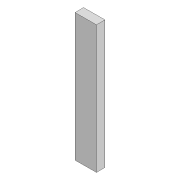
# Autodesk Inventor part: simple_object2
Saved by Autodesk Inventor 2021 (Build 250183000, 183)
## iProperties
Created: 2022-04-11
Part Number: simple_object2
Material: Generic
Document SubType Name: Modeling
Designer: Derm
Density: 1 g/cm^3
Appearance: Default
Author: Derm
Autodesk Inventor part; units mm, degrees
ref_plane "YZ Plane" through (0, 0, 0) normal (1, 0, 0) x (0, 1, 0)
ref_plane "XZ Plane" through (0, 0, 0) normal (0, 1, 0) x (-1, 0, 0)
ref_plane "XY Plane" through (0, 0, 0) normal (0, 0, 1) x (1, 0, 0)
sketch "Sketch1" plane through (0, 0, 0) normal (0, 1, 0) x (-1, 0, 0)
  circle A0 centre (0, 0) radius 1500 construction
  circle A1 centre (0, 0) radius 1500 construction
  circle A2 centre (0, 0) radius 1500 construction
  circle A3 centre (0, 0) radius 1500 construction
  circle A4 centre (0, 0) radius 1500 construction
  circle A5 centre (0, 0) radius 1500 construction
  circle A6 centre (0, 0) radius 1500 construction
  circle A7 centre (0, 0) radius 1500 construction
  circle A8 centre (0, 0) radius 1500 construction
  circle A9 centre (0, 0) radius 1500 construction
  circle A10 centre (0, 0) radius 1500 construction
  circle A11 centre (0, 0) radius 1500 construction
  circle A12 centre (0, 0) radius 1500 construction
  circle A13 centre (0, 0) radius 1500 construction
  circle A14 centre (0, 0) radius 1500 construction
  circle A15 centre (0, 0) radius 1500 construction
  circle A16 centre (50000, 0) radius 38.1
  circle A17 centre (0, 50000) radius 38.1
  circle A18 centre (-50000, 0) radius 38.1
  circle A19 centre (0, -50000) radius 38.1
  line L0 (-250.6668, 98.3166) -> (-249.3219, -101.6789)
  line L1 (-249.3219, -101.6789) -> (250.6668, -98.3166)
  line L2 (250.6668, -98.3166) -> (249.3219, 101.6789)
  line L3 (249.3219, 101.6789) -> (-250.6668, 98.3166)
  line L4 (-250.6668, 98.3166) -> (250.6668, -98.3166) construction
  line L5 (-249.3219, -101.6789) -> (249.3219, 101.6789) construction
  point P0 (1486.3676, 201.7706)
  point P1 (1296.0103, 755.22)
  point P2 (908.3473, 1193.694)
  point P3 (382.3965, 1450.4389)
  point P4 (-201.7706, 1486.3676)
  point P5 (-755.22, 1296.0103)
  point P6 (-1193.694, 908.3473)
  point P7 (-1450.4389, 382.3965)
  point P8 (-1486.3676, -201.7706)
  point P9 (-1296.0103, -755.22)
  point P10 (-908.3473, -1193.694)
  point P11 (-382.3965, -1450.4389)
  point P12 (201.7706, -1486.3676)
  point P13 (755.22, -1296.0103)
  point P14 (1193.694, -908.3473)
  point P15 (1450.4389, -382.3965)
  dimension "d0" = 3000
  dimension "d3" = 360
  dimension "d7" = 50000
  dimension "d10" = 360
  dimension "d12" = 76.2
  dimension "d14" = 200
  dimension "d15" = 500
  constraints: 12 end point, 4 centre point, 4 coincident, 2 midpoint, 2 parallel, 1 perpendicular, 104 other
  measures "d7" distance of point (0, 0) A16.centre
  measures "d12" diameter of A16
  measures "d14" distance of L1.end L2.end
  measures "d15" distance of L0.end L1.end
extrude "Extrusion2" add sketch "Sketch1" along normal mid plane 3000 contours L3 L2 L1 L0
body "Solid2"
